Autodesk Inventor part; units mm, degrees
(part 2 of 2)
sketch "スケッチ14" plane through (0, 0, 1.5) normal (0, 0, 1) x (1, 0, 0)
  circle A0 centre (10.5828, 54.9372) radius 1 projected
  circle A1 centre (-2.2006, -2.6854) radius 1 projected
  circle A2 centre (-2.2006, 50.259) radius 1 projected
  circle A3 centre (10.5828, -7.3636) radius 1 projected
  line L0 (79.4163, 52.576) -> (68.465, 52.576) projected
  arc A4 (66.6353, 53.1986) -> (68.465, 52.576) centre (68.465, 55.576) ccw projected
  line L1 (66.6353, 53.1986) -> (64.0527, 55.1863) projected
  arc A5 (62.8825, 57.5637) -> (64.0527, 55.1863) centre (65.8825, 57.5637) ccw projected
  line L2 (62.8825, 57.5637) -> (62.8825, 60.2904) projected
  arc A6 (63.7611, 62.4117) -> (62.8825, 60.2904) centre (65.8825, 60.2904) ccw projected
  line L3 (63.7611, 62.4117) -> (70.062, 68.7126) projected
  arc A7 (72.1833, 69.5912) -> (70.062, 68.7126) centre (72.1833, 66.5912) ccw projected
  line L4 (72.1833, 69.5912) -> (81.3884, 69.5912) projected
  arc A8 (83.224, 68.9642) -> (81.3884, 69.5912) centre (81.3884, 66.5912) ccw projected
  line L5 (83.224, 68.9642) -> (83.8344, 68.492) projected
  arc A9 (84.9988, 66.1191) -> (83.8344, 68.492) centre (81.9988, 66.1191) ccw projected
  line L6 (84.9988, 66.1191) -> (84.9988, 57.5637) projected
  arc A10 (83.8286, 55.1863) -> (84.9988, 57.5637) centre (81.9988, 57.5637) ccw projected
  line L7 (83.8286, 55.1863) -> (81.246, 53.1986) projected
  arc A11 (79.4163, 52.576) -> (81.246, 53.1986) centre (79.4163, 55.576) ccw projected
  line L8 (68.4658, -5) -> (79.4155, -5) projected
  arc A12 (81.2454, -5.6227) -> (79.4155, -5) centre (79.4155, -8) ccw projected
  line L9 (81.2454, -5.6227) -> (83.8287, -7.6112) projected
  arc A13 (84.9988, -9.9885) -> (83.8287, -7.6112) centre (81.9988, -9.9885) ccw projected
  line L10 (84.9988, -9.9885) -> (84.9988, -18.6112) projected
  arc A14 (83.8344, -20.9841) -> (84.9988, -18.6112) centre (81.9988, -18.6112) ccw projected
  line L11 (83.8344, -20.9841) -> (83.224, -21.4563) projected
  arc A15 (81.3884, -22.0833) -> (83.224, -21.4563) centre (81.3884, -19.0833) ccw projected
  line L12 (81.3884, -22.0833) -> (72.1833, -22.0833) projected
  arc A16 (70.062, -21.2047) -> (72.1833, -22.0833) centre (72.1833, -19.0833) ccw projected
  line L13 (70.062, -21.2047) -> (63.7611, -14.9038) projected
  arc A17 (62.8825, -12.7825) -> (63.7611, -14.9038) centre (65.8825, -12.7825) ccw projected
  line L14 (62.8825, -12.7825) -> (62.8825, -9.9885) projected
  arc A18 (64.0526, -7.6112) -> (62.8825, -9.9885) centre (65.8825, -9.9885) ccw projected
  line L15 (64.0526, -7.6112) -> (66.6359, -5.6227) projected
  arc A19 (68.4658, -5) -> (66.6359, -5.6227) centre (68.4658, -8) ccw projected
  arc A20 (57.5082, 18.2012) -> (60.5082, 21.2012) centre (57.5082, 21.2012) ccw projected
  line L16 (60.5082, 21.2012) -> (60.5082, 24.5012) projected
  ellipse E0 centre (57.0082, 24.5012) end of major axis (53.5082, 24.5012) minor radius 3.5 (60.5082, 24.5012) -> (53.6027, 25.3089) ccw projected
  arc A21 (50.6837, 23.0012) -> (53.6027, 25.3089) centre (50.6837, 26.0012) ccw projected
  line L17 (50.6837, 23.0012) -> (5, 23.0012) projected
  line L18 (5, 23.0012) -> (5, 24.5012) projected
  ellipse E1 centre (2.5, 24.5012) end of major axis (5, 24.5012) minor radius 2.5 (5, 24.5012) -> (2.5, 27.0012) ccw projected
  line L19 (2.5, 27.0012) -> (1, 27.0012) projected
  arc A22 (0, 28.0012) -> (1, 27.0012) centre (1, 28.0012) ccw projected
  line L20 (0, 28.0012) -> (0, 44.576) projected
  arc A23 (3, 47.576) -> (0, 44.576) centre (3, 44.576) ccw projected
  line L21 (3, 47.576) -> (87, 47.576) projected
  arc A24 (90, 44.576) -> (87, 47.576) centre (87, 44.576) ccw projected
  line L22 (90, 44.576) -> (90, 29.7874) projected
  ellipse E2 centre (87, 29.7874) end of major axis (87, 26.7874) minor radius 3 (87, 26.7874) -> (90, 29.7874) ccw projected
  ellipse E3 centre (87.471, 23.7874) end of major axis (84.4343, 23.7874) minor radius 3.0367 (87, 26.7874) -> (85, 25.5526) ccw projected
  line L23 (85, 25.5526) -> (85, 22.0222) projected
  ellipse E4 centre (87.471, 23.7874) end of major axis (84.4343, 23.7874) minor radius 3.0367 (85, 22.0222) -> (87, 20.7874) ccw projected
  arc A25 (90, 17.7874) -> (87, 20.7874) centre (87, 17.7874) ccw projected
  line L24 (90, 17.7874) -> (90, 3) projected
  arc A26 (87, 0) -> (90, 3) centre (87, 3) ccw projected
  line L25 (87, 0) -> (3, 0) projected
  arc A27 (0, 3) -> (3, 0) centre (3, 3) ccw projected
  line L26 (0, 3) -> (0, 15.2012) projected
  arc A28 (3, 18.2012) -> (0, 15.2012) centre (3, 15.2012) ccw projected
  line L27 (3, 18.2012) -> (57.5082, 18.2012) projected
  line L28 (40.3806, 69.6542) -> (53.3375, 56.6973) projected
  arc A29 (51.2162, 51.576) -> (53.3375, 56.6973) centre (51.2162, 54.576) ccw projected
  line L29 (51.2162, 51.576) -> (25.3023, 51.576) projected
  arc A30 (23.181, 56.6973) -> (25.3023, 51.576) centre (25.3023, 54.576) ccw projected
  line L30 (23.181, 56.6973) -> (36.1379, 69.6542) projected
  arc A31 (40.3806, 69.6542) -> (36.1379, 69.6542) centre (38.2592, 67.5329) ccw projected
  line L31 (35.8537, -22.3623) -> (22.6127, -9.1213) projected
  arc A32 (24.734, -4) -> (22.6127, -9.1213) centre (24.734, -7) ccw projected
  line L32 (24.734, -4) -> (51.2161, -4) projected
  arc A33 (53.3374, -9.1213) -> (51.2161, -4) centre (51.2161, -7) ccw projected
  line L33 (53.3374, -9.1213) -> (40.0964, -22.3623) projected
  arc A34 (35.8537, -22.3623) -> (40.0964, -22.3623) centre (37.975, -20.241) ccw projected
  arc A35 (46.9123, -44.2207) -> (49.0336, -45.0993) centre (49.0336, -42.0993) ccw projected
  line L34 (49.0336, -45.0993) -> (56.8481, -45.0993) projected
  arc A36 (56.8481, -45.0993) -> (58.9694, -44.2207) centre (56.8481, -42.0993) ccw projected
  line L35 (59.3492, -43.8408) -> (58.9694, -44.2207) projected
  arc A37 (59.3492, -43.8408) -> (60.2081, -41.3754) centre (57.2279, -41.7195) ccw projected
  arc A38 (70.0856, -29.1585) -> (60.2081, -41.3754) centre (71.1407, -40.1131) ccw projected
  ellipse E5 centre (71.1407, -40.1131) end of major axis (60.1355, -40.1131) minor radius 11.0053 (73.7648, -29.4252) -> (70.0856, -29.1585) ccw projected
  line L36 (73.7648, -29.4252) -> (78.0095, -28.8072) projected
  line L37 (78.0095, -28.8072) -> (88.1117, -26.0409) projected
  arc A39 (88.1117, -26.0409) -> (90.2129, -23.9396) centre (87.3194, -23.1474) ccw projected
  ellipse E6 centre (96, -25.5238) end of major axis (102, -25.5238) minor radius 6 (92.5, -20.6504) -> (90.2129, -23.9396) ccw projected
  ellipse E7 centre (89, -15.777) end of major axis (83, -15.777) minor radius 6 (92.5, -20.6504) -> (95, -15.777) ccw projected
  line L38 (95, -15.777) -> (95, 63.3506) projected
  ellipse E8 centre (89, 63.3506) end of major axis (89, 69.3506) minor radius 6 (95, 63.3506) -> (92.5, 68.224) ccw projected
  ellipse E9 centre (96, 73.0974) end of major axis (96, 67.0974) minor radius 6 (90.2129, 71.5134) -> (92.5, 68.224) ccw projected
  arc A40 (90.2129, 71.5134) -> (88.1122, 73.6148) centre (87.3193, 70.7215) ccw projected
  line L39 (88.1122, 73.6148) -> (78.0106, 76.3832) projected
  line L40 (78.0106, 76.3832) -> (74.0275, 76.9631) projected
  line L41 (74.0275, 76.9631) -> (69.9975, 76.6465) projected
  arc A41 (60.1193, 89.0223) -> (69.9975, 76.6465) centre (71.1407, 87.6892) ccw projected
  arc A42 (60.1193, 89.0223) -> (59.2623, 91.5038) centre (57.141, 89.3825) ccw projected
  line L42 (58.9694, 91.7968) -> (59.2623, 91.5038) projected
  arc A43 (58.9694, 91.7968) -> (56.8481, 92.6754) centre (56.8481, 89.6754) ccw projected
  line L43 (56.8481, 92.6754) -> (49.0349, 92.6754) projected
  arc A44 (49.0349, 92.6754) -> (46.9136, 91.7968) centre (49.0349, 89.6754) ccw projected
  line L44 (46.9136, 91.7968) -> (17.6928, 62.576) projected
  line L45 (-5, 52.5748) -> (17.6928, 62.576) projected
  line L46 (-5, 52.5748) -> (-5, -5.0012) projected
  line L47 (-5, -5.0012) -> (-4.9972, -5.0012) projected
  line L48 (17.6898, -14.9981) -> (-4.9972, -5.0012) projected
  line L49 (17.6898, -14.9981) -> (46.9123, -44.2207) projected
  circle A45 centre (58.0239, -41.4919) radius 0.75 projected
  circle A46 centre (58.0239, 89.068) radius 0.75 projected
  circle A47 centre (2.5, 24.5003) radius 1 projected
  circle A48 centre (57.0082, 24.5003) radius 1 projected
  circle A49 centre (57.8825, 59.9352) radius 1.05 projected
  circle A50 centre (43.3868, 74.4309) radius 1.05 projected
  circle A51 centre (72.5196, 74.5724) radius 1.05 projected
  circle A52 centre (87.471, 23.7874) radius 1 projected
  circle A53 centre (89.9993, 59.9351) radius 1.05 projected
  circle A54 centre (72.5196, -26.9962) radius 1.05 projected
  circle A55 centre (57.8825, -12.3591) radius 1.05 projected
  circle A56 centre (43.3868, -26.8548) radius 1.05 projected
  circle A57 centre (89.9988, -12.3606) radius 1.05 projected
  line L50 (55.7611, 65.5921) -> (49.0436, 72.3096) projected
  arc A58 (49.0436, 76.5523) -> (49.0436, 72.3096) centre (51.1649, 74.4309) ccw projected
  line L51 (49.0436, 76.5523) -> (53.9214, 81.4301) projected
  arc A59 (58.1641, 81.4301) -> (53.9214, 81.4301) centre (56.0428, 79.3088) ccw projected
  line L52 (58.1641, 81.4301) -> (64.8816, 74.7126) projected
  arc A60 (64.8816, 70.4699) -> (64.8816, 74.7126) centre (62.7603, 72.5912) ccw projected
  line L53 (64.8816, 70.4699) -> (60.0038, 65.5921) projected
  arc A61 (55.7611, 65.5921) -> (60.0038, 65.5921) centre (57.8825, 67.7134) ccw projected
  line L54 (60.0038, -18.016) -> (64.9498, -22.962) projected
  arc A62 (64.9498, -27.2047) -> (64.9498, -22.962) centre (62.8285, -25.0833) ccw projected
  line L55 (64.9498, -27.2047) -> (58.2323, -33.9222) projected
  arc A63 (53.9897, -33.9222) -> (58.2323, -33.9222) centre (56.111, -31.8009) ccw projected
  line L56 (53.9897, -33.9222) -> (49.0436, -28.9761) projected
  arc A64 (49.0436, -24.7335) -> (49.0436, -28.9761) centre (51.1649, -26.8548) ccw projected
  line L57 (49.0436, -24.7335) -> (55.7611, -18.016) projected
  arc A65 (60.0038, -18.016) -> (55.7611, -18.016) centre (57.8825, -20.1373) ccw projected
  line L58 (5, 23.0012) -> (5, 18.2012)
  point P0 (0, 0)
  constraints: 2 end point, 1 perpendicular, 1 point on line, 10 other
extrude "押し出し13" cut sketch "スケッチ14" against normal blind 10 contours L27 L58 L17 A21 E0 L16 A20
fillet "フィレット7" radius 2 1 edges at (5, 18.2012, 0.75)
equation "\"d16\" = d15"
